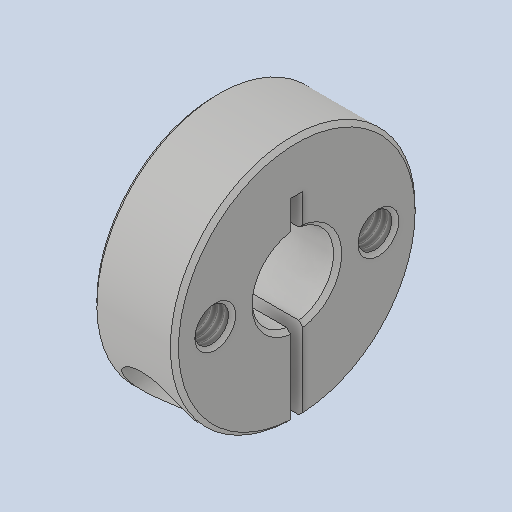
# Autodesk Inventor part: SSCSW10-10b
Saved by Autodesk Inventor 2025.2 (Build 292293000, 293)
## iProperties
Created: 2024-07-22
Part Number: SSCSW10-10b
Material: Generic
Catalog Web Link: www.cadenas.de
Description: SCSW, PSCSW, SSCSW, SCSWA, SCSWAW-b-Set Collars - Slit 2 Hole/2 Tap - Standard Type - 2 Tap Type
Vendor: MISUMI
Document SubType Name: Modeling
Designer: psAdmin
Manufacturer: MISUMI
Mass: 5.30911 g
Surface Area: 31.0437 cm^2
Volume: 5.30911 cm^3
Density: 1 g/cm^3
Appearance: PSOLRGB-175-175-175
Category: PARTsolutions
Company: MISUMI
PSOL_IDENT_0: {$CADENAS_DATA/23d-libs/misumi/metric/03_set_collars/scsw_b.prj},202 {VTYP=3D},{NB=SSCSW10-10b},{LIN
PSOL_IDENT_1: A=SSCSW10-10b},{NN=SCSW, PSCSW, SSCSW, SCSWA, SCSWAW-b},{DATE=04.10.2021 04:21:03},{GEOMDATE=15.09.2
PSOL_IDENT_2: 021 06:01:21},{VERSION=},{LINEID=60},{WBVAR=MAT,ST,BS},{WBNUMERIC=BS}  {NB=SSCSW10-10b},{LINA=SSCSW1
PSOL_IDENT_3: 0-10b},{KT=DUMMY},{PN=SSCSW10-10},{TYPE=SSCSW},{MAT=304},{MATA='1045','S45C Equivalent','304','SUS30
PSOL_IDENT_4: 4 Equivalent','2017','2017 Aluminum Alloy'},{ST=-},{AC=Hexagon Socket Head Set Screw 1 Pc. (304 Stai
PSOL_IDENT_5: nless Steel) },{D=10},{BS=10},{B1=8,10,12},{D1=30},{M=M4},{THMD=4},{THDMIN=3.242},{ST0='-','-'},{DD=
PSOL_IDENT_6: 4.5},{R=3.75},{W=1.5},{X=9.0},{Y=5.0},{Z=8~10},{S=5.5},{P=20},{C=0.5},{L=10},{M1=M5},{ZZ=9},{THMD1=5
PSOL_IDENT_7: },{THDMIN1=4.134}
NB: SSCSW10-10b
NN: SCSW, PSCSW, SSCSW, SCSWA, SCSWAW-b
NT: Set Collars - Slit 2 Hole/2 Tap - Standard Type - 2 Tap Type
NBSYN: $PN.b
LINA: SSCSW10-10b
CATALOG: Misumi
PN: SSCSW10-10
MAT: SUS304 Equivalent
ST: -
AC: Hexagon Socket Head Set Screw 1 Pc. (304 Stainless Steel)
D: 10
BS: 10
D1: 30
M: M4
DD: 4.5
R: 3.75
W: 1.5
X: 9
Y: 5
Z: 8~10
S: 5.5
P: 20
M1: M5
SUPPLIER: MISUMI
ARTICLENO: SSCSW10-10b
BOMINFO: SSCSW10-10b
CREATOR: CADENAS GmbH
Title: SSCSW10-10b
Author: Cadenas PARTsolutions
Comments: Set Collars - Slit 2 Hole/2 Tap - Standard Type - 2 Tap Type
Autodesk Inventor part; units mm, degrees
sketch "Sketch_1" plane through (0, 0, 0) normal (0, 0, 1) x (1, 0, 0)
  line L0 (5, 0) -> (-5, 0)
  line L1 (-5, 14.5) -> (-5, 5.5)
  line L2 (-5, 5.5) -> (-4.5, 5)
  line L3 (-4.5, 5) -> (4.5, 5)
  line L4 (4.5, 5) -> (5, 5.5)
  line L5 (5, 5.5) -> (5, 14.5)
  line L6 (5, 14.5) -> (4.5, 15)
  line L7 (4.5, 15) -> (-4.5, 15)
  line L8 (-4.5, 15) -> (-5, 14.5)
  constraints: 18 end point
revolve "Revolution1" add sketch "Sketch_1" angle 360 about axis through (5, 0, 0) along (1, 0, 0)
sketch "Sketch_2" plane through (0, 0, 0) normal (1, 0, 0) x (0, 1, 0)
  line L0 (-15, 0.75) -> (-15, -0.75)
  line L1 (-15, -0.75) -> (9, -0.75)
  line L2 (9, -0.75) -> (9, 0.75)
  line L3 (9, 0.75) -> (-15, 0.75)
  constraints: 8 end point
extrude "Extrusion1" cut sketch "Sketch_2" along normal mid plane 10
sketch "Sketch_3" plane through (0, 0, 0) normal (1, 0, 0) x (0, 1, 0)
  line L0 (-9, 15) -> (-9, 0)
  line L1 (-9, 0) -> (-11.25, 0)
  line L2 (-11.25, 0) -> (-11.25, 5)
  line L3 (-11.25, 5) -> (-12.75, 5)
  line L4 (-12.75, 5) -> (-12.75, 15)
  line L5 (-12.75, 15) -> (-9, 15)
  line L6 (-9, 15) -> (-9, 0)
  constraints: 14 end point
revolve "Revolution2" cut sketch "Sketch_3" angle 360 about axis through (0, -9, 15) along (0, 0, 1)
sketch "Sketch_4" plane through (0, 0, 0) normal (1, 0, 0) x (0, 1, 0)
  line L0 (-9, -14.25) -> (-9, -0.75)
  line L1 (-9, -0.75) -> (-7, -0.75)
  line L2 (-7, -0.75) -> (-7.379, -1.129)
  line L3 (-7.379, -1.129) -> (-7.379, -14.25)
  line L4 (-7.379, -14.25) -> (-9, -14.25)
  line L5 (-9, -14.25) -> (-9, -0.75)
  constraints: 12 end point
revolve "Revolution3" cut sketch "Sketch_4" angle 360 about axis through (0, -9, -14.25) along (0, 0, -1)
thread "Thread1" size "M4x0.7" class "6H" standard "ISO Metric profile" length 12.1375
sketch "Sketch_7" plane through (0, 0, -10) normal (0, 0, 1) x (1, 0, 0)
  line L0 (5, 0) -> (-5, 0)
  line L1 (-5, 0) -> (-5, 2.5)
  line L2 (-5, 2.5) -> (-4.567, 2.067)
  line L3 (-4.567, 2.067) -> (4.567, 2.067)
  line L4 (4.567, 2.067) -> (5, 2.5)
  line L5 (5, 2.5) -> (5, 0)
  line L6 (5, 0) -> (-5, 0)
  constraints: 14 end point
revolve "Revolution4" cut sketch "Sketch_7" angle 360 about axis through (5, 0, -10) along (1, 0, 0)
thread "Thread2" size "M5x0.8" class "6H" standard "ISO Metric profile" full length
sketch "Sketch_8" plane through (0, 0, 10) normal (0, 0, 1) x (1, 0, 0)
  line L0 (5, 0) -> (-5, 0)
  line L1 (-5, 0) -> (-5, 2.5)
  line L2 (-5, 2.5) -> (-4.567, 2.067)
  line L3 (-4.567, 2.067) -> (4.567, 2.067)
  line L4 (4.567, 2.067) -> (5, 2.5)
  line L5 (5, 2.5) -> (5, 0)
  line L6 (5, 0) -> (-5, 0)
  constraints: 14 end point
revolve "Revolution5" cut sketch "Sketch_8" angle 360 about axis through (5, 0, 10) along (1, 0, 0)
thread "Thread3" size "M5x0.8" class "6H" standard "ISO Metric profile" full length
ref_plane "body_screw_XY" through (0, -9, 5) normal (0, 0, 1) x (1, 0, 0)
ref_plane "body_screw_YZ" through (0, -9, 5) normal (1, 0, 0) x (0, 1, 0)
ref_plane "body_screw_ZX" through (0, -9, 5) normal (0, 1, 0) x (0, 0, 1)
body "Solid1"
